Autodesk Fusion 360 part; units mm, degrees
(part 5 of 7)
  line L387 (58.55, -43.6287) -> (58.588, -43.6922)
  line L388 (58.588, -43.6922) -> (58.628, -43.7538)
  line L389 (58.628, -43.7538) -> (58.6706, -43.8129)
  line L390 (58.6706, -43.8129) -> (58.7169, -43.8682)
  line L391 (58.7169, -43.8682) -> (59.0326, -44.185)
  line L392 (59.0326, -44.185) -> (58.8812, -44.34)
  line L393 (58.8812, -44.34) -> (58.734, -44.4991)
  line L394 (58.734, -44.4991) -> (58.5912, -44.6621)
  line L395 (58.5912, -44.6621) -> (58.4529, -44.8289)
  line L396 (58.4529, -44.8289) -> (58.1048, -44.548)
  line L397 (58.1048, -44.548) -> (58.0449, -44.5077)
  line L398 (58.0449, -44.5077) -> (57.9817, -44.4716)
  line L399 (57.9817, -44.4716) -> (57.9163, -44.4382)
  line L400 (57.9163, -44.4382) -> (57.8491, -44.4071)
  line L401 (57.8491, -44.4071) -> (57.7804, -44.3781)
  line L402 (57.7804, -44.3781) -> (57.7102, -44.3509)
  line L403 (57.7102, -44.3509) -> (57.6387, -44.3254)
  line L404 (57.6387, -44.3254) -> (57.566, -44.3017)
  line L405 (57.566, -44.3017) -> (57.4922, -44.2795)
  line L406 (57.4922, -44.2795) -> (57.4173, -44.2588)
  line L407 (57.4173, -44.2588) -> (57.3414, -44.2397)
  line L408 (57.3414, -44.2397) -> (57.2644, -44.222)
  line L409 (57.2644, -44.222) -> (57.1855, -44.3275)
  line L410 (57.1855, -44.3275) -> (57.108, -44.4341)
  line L411 (57.108, -44.4341) -> (57.032, -44.5418)
  line L412 (57.032, -44.5418) -> (57.0726, -44.6095)
  line L413 (57.0726, -44.6095) -> (57.1143, -44.6758)
  line L414 (57.1143, -44.6758) -> (57.1571, -44.7407)
  line L415 (57.1571, -44.7407) -> (57.201, -44.804)
  line L416 (57.201, -44.804) -> (57.2461, -44.8658)
  line L417 (57.2461, -44.8658) -> (57.2924, -44.9259)
  line L418 (57.2924, -44.9259) -> (57.3399, -44.9843)
  line L419 (57.3399, -44.9843) -> (57.3888, -45.0407)
  line L420 (57.3888, -45.0407) -> (57.4392, -45.095)
  line L421 (57.4392, -45.095) -> (57.4911, -45.1469)
  line L422 (57.4911, -45.1469) -> (57.545, -45.1958)
  line L423 (57.545, -45.1958) -> (57.6018, -45.2403)
  line L424 (57.6018, -45.2403) -> (57.9765, -45.4845)
  line L425 (57.9765, -45.4845) -> (57.8606, -45.6677)
  line L426 (57.8606, -45.6677) -> (57.7497, -45.8538)
  line L427 (57.7497, -45.8538) -> (57.6439, -46.0429)
  line L428 (57.6439, -46.0429) -> (57.5433, -46.2348)
  line L429 (57.5433, -46.2348) -> (57.1444, -46.0325)
  line L430 (57.1444, -46.0325) -> (57.0775, -46.0056)
  line L431 (57.0775, -46.0056) -> (57.0082, -45.9834)
  line L432 (57.0082, -45.9834) -> (56.9372, -45.9643)
  line L433 (56.9372, -45.9643) -> (56.8651, -45.9479)
  line L434 (56.8651, -45.9479) -> (56.7918, -45.9337)
  line L435 (56.7918, -45.9337) -> (56.7175, -45.9217)
  line L436 (56.7175, -45.9217) -> (56.6423, -45.9117)
  line L437 (56.6423, -45.9117) -> (56.5662, -45.9035)
  line L438 (56.5662, -45.9035) -> (56.4894, -45.8972)
  line L439 (56.4894, -45.8972) -> (56.4118, -45.8926)
  line L440 (56.4118, -45.8926) -> (56.3336, -45.8896)
  line L441 (56.3336, -45.8896) -> (56.2547, -45.8883)
  line L442 (56.2547, -45.8883) -> (56.1994, -46.0079)
  line L443 (56.1994, -46.0079) -> (56.1458, -46.1283)
  line L444 (56.1458, -46.1283) -> (56.0939, -46.2495)
  line L445 (56.0939, -46.2495) -> (56.1476, -46.3073)
  line L446 (56.1476, -46.3073) -> (56.2022, -46.3634)
  line L447 (56.2022, -46.3634) -> (56.2575, -46.418)
  line L448 (56.2575, -46.418) -> (56.3137, -46.4708)
  line L449 (56.3137, -46.4708) -> (56.3706, -46.5219)
  line L450 (56.3706, -46.5219) -> (56.4284, -46.5711)
  line L451 (56.4284, -46.5711) -> (56.487, -46.6182)
  line L452 (56.487, -46.6182) -> (56.5465, -46.6633)
  line L453 (56.5465, -46.6633) -> (56.6071, -46.7059)
  line L454 (56.6071, -46.7059) -> (56.6687, -46.7458)
  line L455 (56.6687, -46.7458) -> (56.7316, -46.7825)
  line L456 (56.7316, -46.7825) -> (56.7964, -46.8142)
  line L457 (56.7964, -46.8142) -> (57.2136, -46.9753)
  line L458 (57.2136, -46.9753) -> (57.1384, -47.1784)
  line L459 (57.1384, -47.1784) -> (57.0686, -47.3836)
  line L460 (57.0686, -47.3836) -> (57.0045, -47.5906)
  line L461 (57.0045, -47.5906) -> (56.9459, -47.7992)
  line L462 (56.9459, -47.7992) -> (56.5137, -47.6842)
  line L463 (56.5137, -47.6842) -> (56.4426, -47.6718)
  line L464 (56.4426, -47.6718) -> (56.3702, -47.6645)
  line L465 (56.3702, -47.6645) -> (56.2969, -47.6606)
  line L466 (56.2969, -47.6606) -> (56.2228, -47.6595)
  line L467 (56.2228, -47.6595) -> (56.1482, -47.6609)
  line L468 (56.1482, -47.6609) -> (56.0731, -47.6646)
  line L469 (56.0731, -47.6646) -> (55.9974, -47.6705)
  line L470 (55.9974, -47.6705) -> (55.9213, -47.6783)
  line L471 (55.9213, -47.6783) -> (55.8449, -47.6881)
  line L472 (55.8449, -47.6881) -> (55.768, -47.6997)
  line L473 (55.768, -47.6997) -> (55.6909, -47.713)
  line L474 (55.6909, -47.713) -> (55.6134, -47.7282)
  line L475 (55.6134, -47.7282) -> (55.5842, -47.8567)
  line L476 (55.5842, -47.8567) -> (55.5568, -47.9856)
  line L477 (55.5568, -47.9856) -> (55.5312, -48.1149)
  line L478 (55.5312, -48.1149) -> (55.5958, -48.1602)
  line L479 (55.5958, -48.1602) -> (55.6609, -48.2038)
  line L480 (55.6609, -48.2038) -> (55.7263, -48.2457)
  line L481 (55.7263, -48.2457) -> (55.7922, -48.2857)
  line L482 (55.7922, -48.2857) -> (55.8585, -48.3238)
  line L483 (55.8585, -48.3238) -> (55.9253, -48.3599)
  line L484 (55.9253, -48.3599) -> (55.9924, -48.3938)
  line L485 (55.9924, -48.3938) -> (56.06, -48.4255)
  line L486 (56.06, -48.4255) -> (56.1281, -48.4546)
  line L487 (56.1281, -48.4546) -> (56.1967, -48.4809)
  line L488 (56.1967, -48.4809) -> (56.2658, -48.5037)
  line L489 (56.2658, -48.5037) -> (56.3358, -48.5212)
  line L490 (56.3358, -48.5212) -> (56.7774, -48.592)
  line L491 (56.7774, -48.592) -> (56.746, -48.8064)
  line L492 (56.746, -48.8064) -> (56.7205, -49.0216)
  line L493 (56.7205, -49.0216) -> (56.7007, -49.2373)
  line L494 (56.7007, -49.2373) -> (56.6868, -49.4536)
  line L495 (56.6868, -49.4536) -> (56.2402, -49.431)
  line L496 (56.2402, -49.431) -> (56.1681, -49.4336)
  line L497 (56.1681, -49.4336) -> (56.0957, -49.4415)
  line L498 (56.0957, -49.4415) -> (56.0232, -49.4529)
  line L499 (56.0232, -49.4529) -> (55.9505, -49.4673)
  line L500 (55.9505, -49.4673) -> (55.8778, -49.4842)
  line L501 (55.8778, -49.4842) -> (55.8051, -49.5034)
  line L502 (55.8051, -49.5034) -> (55.7323, -49.5249)
  line L503 (55.7323, -49.5249) -> (55.6595, -49.5483)
  line L504 (55.6595, -49.5483) -> (55.5867, -49.5738)
  line L505 (55.5867, -49.5738) -> (55.514, -49.6011)
  line L506 (55.514, -49.6011) -> (55.4413, -49.6302)
  line L507 (55.4413, -49.6302) -> (55.3687, -49.6611)
  line L508 (55.3687, -49.6611) -> (55.3668, -49.7929)
  line L509 (55.3668, -49.7929) -> (55.3668, -49.9247)
  line L510 (55.3668, -49.9247) -> (55.3687, -50.0565)
  line L511 (55.3687, -50.0565) -> (55.4413, -50.0874)
  line L512 (55.4413, -50.0874) -> (55.514, -50.1166)
  line L513 (55.514, -50.1166) -> (55.5867, -50.1439)
  line L514 (55.5867, -50.1439) -> (55.6595, -50.1693)
  line L515 (55.6595, -50.1693) -> (55.7323, -50.1928)
  line L516 (55.7323, -50.1928) -> (55.8051, -50.2142)
  line L517 (55.8051, -50.2142) -> (55.8778, -50.2335)
  line L518 (55.8778, -50.2335) -> (55.9505, -50.2504)
  line L519 (55.9505, -50.2504) -> (56.0232, -50.2647)
  line L520 (56.0232, -50.2647) -> (56.0957, -50.2762)
  line L521 (56.0957, -50.2762) -> (56.1681, -50.2841)
  line L522 (56.1681, -50.2841) -> (56.2402, -50.2867)
  line L523 (56.2402, -50.2867) -> (56.6868, -50.2641)
  line L524 (56.6868, -50.2641) -> (56.7007, -50.4803)
  line L525 (56.7007, -50.4803) -> (56.7205, -50.6961)
  line L526 (56.7205, -50.6961) -> (56.746, -50.9113)
  line L527 (56.746, -50.9113) -> (56.7774, -51.1257)
  line L528 (56.7774, -51.1257) -> (56.3358, -51.1964)
  line L529 (56.3358, -51.1964) -> (56.2658, -51.214)
  line L530 (56.2658, -51.214) -> (56.1967, -51.2368)
  line L531 (56.1967, -51.2368) -> (56.1281, -51.263)
  line L532 (56.1281, -51.263) -> (56.06, -51.2922)
  line L533 (56.06, -51.2922) -> (55.9924, -51.3238)
  line L534 (55.9924, -51.3238) -> (55.9253, -51.3578)
  line L535 (55.9253, -51.3578) -> (55.8585, -51.3939)
  line L536 (55.8585, -51.3939) -> (55.7922, -51.432)
  line L537 (55.7922, -51.432) -> (55.7263, -51.472)
  line L538 (55.7263, -51.472) -> (55.6609, -51.5138)
  line L539 (55.6609, -51.5138) -> (55.5958, -51.5574)
  line L540 (55.5958, -51.5574) -> (55.5312, -51.6028)
  line L541 (55.5312, -51.6028) -> (55.5568, -51.7321)
  line L542 (55.5568, -51.7321) -> (55.5842, -51.861)
  line L543 (55.5842, -51.861) -> (55.6134, -51.9895)
  line L544 (55.6134, -51.9895) -> (55.6909, -52.0046)
  line L545 (55.6909, -52.0046) -> (55.768, -52.018)
  line L546 (55.768, -52.018) -> (55.8449, -52.0296)
  line L547 (55.8449, -52.0296) -> (55.9213, -52.0394)
  line L548 (55.9213, -52.0394) -> (55.9974, -52.0472)
  line L549 (55.9974, -52.0472) -> (56.0731, -52.053)
  line L550 (56.0731, -52.053) -> (56.1482, -52.0567)
  line L551 (56.1482, -52.0567) -> (56.2228, -52.0582)
  line L552 (56.2228, -52.0582) -> (56.2969, -52.0571)
  line L553 (56.2969, -52.0571) -> (56.3702, -52.0532)
  line L554 (56.3702, -52.0532) -> (56.4426, -52.0459)
  line L555 (56.4426, -52.0459) -> (56.5137, -52.0335)
  line L556 (56.5137, -52.0335) -> (56.9459, -51.9185)
  line L557 (56.9459, -51.9185) -> (57.0045, -52.1271)
  line L558 (57.0045, -52.1271) -> (57.0686, -52.3341)
  line L559 (57.0686, -52.3341) -> (57.1384, -52.5392)
  line L560 (57.1384, -52.5392) -> (57.2136, -52.7424)
  line L561 (57.2136, -52.7424) -> (56.7964, -52.9034)
  line L562 (56.7964, -52.9034) -> (56.7316, -52.9352)
  line L563 (56.7316, -52.9352) -> (56.6687, -52.9718)
  line L564 (56.6687, -52.9718) -> (56.6071, -53.0118)
  line L565 (56.6071, -53.0118) -> (56.5465, -53.0544)
  line L566 (56.5465, -53.0544) -> (56.487, -53.0994)
  line L567 (56.487, -53.0994) -> (56.4284, -53.1466)
  line L568 (56.4284, -53.1466) -> (56.3706, -53.1958)
  line L569 (56.3706, -53.1958) -> (56.3137, -53.2468)
  line L570 (56.3137, -53.2468) -> (56.2575, -53.2997)
  line L571 (56.2575, -53.2997) -> (56.2022, -53.3542)
  line L572 (56.2022, -53.3542) -> (56.1476, -53.4104)
  line L573 (56.1476, -53.4104) -> (56.0939, -53.4682)
  line L574 (56.0939, -53.4682) -> (56.1458, -53.5893)
  line L575 (56.1458, -53.5893) -> (56.1994, -53.7097)
  line L576 (56.1994, -53.7097) -> (56.2547, -53.8294)
  line L577 (56.2547, -53.8294) -> (56.3336, -53.828)
  line L578 (56.3336, -53.828) -> (56.4118, -53.8251)
  line L579 (56.4118, -53.8251) -> (56.4894, -53.8205)
  line L580 (56.4894, -53.8205) -> (56.5662, -53.8141)
  line L581 (56.5662, -53.8141) -> (56.6423, -53.806)
  line L582 (56.6423, -53.806) -> (56.7175, -53.7959)
  line L583 (56.7175, -53.7959) -> (56.7918, -53.7839)
  line L584 (56.7918, -53.7839) -> (56.8651, -53.7698)
  line L585 (56.8651, -53.7698) -> (56.9372, -53.7534)
  line L586 (56.9372, -53.7534) -> (57.0082, -53.7343)
  line L587 (57.0082, -53.7343) -> (57.0775, -53.7121)
  line L588 (57.0775, -53.7121) -> (57.1444, -53.6852)
  line L589 (57.1444, -53.6852) -> (57.5433, -53.4828)
  line L590 (57.5433, -53.4828) -> (57.6439, -53.6747)
  line L591 (57.6439, -53.6747) -> (57.7497, -53.8638)
  line L592 (57.7497, -53.8638) -> (57.8606, -54.05)
  line L593 (57.8606, -54.05) -> (57.9765, -54.2331)
  line L594 (57.9765, -54.2331) -> (57.6018, -54.4773)
  line L595 (57.6018, -54.4773) -> (57.545, -54.5219)
  line L596 (57.545, -54.5219) -> (57.4911, -54.5708)
  line L597 (57.4911, -54.5708) -> (57.4392, -54.6227)
  line L598 (57.4392, -54.6227) -> (57.3888, -54.677)
  line L599 (57.3888, -54.677) -> (57.3399, -54.7334)
  line L600 (57.3399, -54.7334) -> (57.2924, -54.7917)
  line L601 (57.2924, -54.7917) -> (57.2461, -54.8518)
  line L602 (57.2461, -54.8518) -> (57.201, -54.9136)
  line L603 (57.201, -54.9136) -> (57.1571, -54.977)
  line L604 (57.1571, -54.977) -> (57.1143, -55.0418)
  line L605 (57.1143, -55.0418) -> (57.0726, -55.1081)
  line L606 (57.0726, -55.1081) -> (57.032, -55.1758)
  line L607 (57.032, -55.1758) -> (57.108, -55.2835)
  line L608 (57.108, -55.2835) -> (57.1855, -55.3902)
  line L609 (57.1855, -55.3902) -> (57.2644, -55.4957)
  line L610 (57.2644, -55.4957) -> (57.3414, -55.478)
  line L611 (57.3414, -55.478) -> (57.4173, -55.4588)
  line L612 (57.4173, -55.4588) -> (57.4922, -55.4382)
  line L613 (57.4922, -55.4382) -> (57.566, -55.416)
  line L614 (57.566, -55.416) -> (57.6387, -55.3922)
  line L615 (57.6387, -55.3922) -> (57.7102, -55.3668)
  line L616 (57.7102, -55.3668) -> (57.7804, -55.3396)
  line L617 (57.7804, -55.3396) -> (57.8491, -55.3105)
  line L618 (57.8491, -55.3105) -> (57.9163, -55.2794)
  line L619 (57.9163, -55.2794) -> (57.9817, -55.2461)
  line L620 (57.9817, -55.2461) -> (58.0449, -55.2099)
  line L621 (58.0449, -55.2099) -> (58.1048, -55.1697)
  line L622 (58.1048, -55.1697) -> (58.4529, -54.8888)
  line L623 (58.4529, -54.8888) -> (58.5912, -55.0556)
  line L624 (58.5912, -55.0556) -> (58.734, -55.2186)
  line L625 (58.734, -55.2186) -> (58.8812, -55.3776)
  line L626 (58.8812, -55.3776) -> (59.0326, -55.5326)
  line L627 (59.0326, -55.5326) -> (58.7169, -55.8494)
  line L628 (58.7169, -55.8494) -> (58.6706, -55.9048)
  line L629 (58.6706, -55.9048) -> (58.628, -55.9639)
  line L630 (58.628, -55.9639) -> (58.588, -56.0254)
  line L631 (58.588, -56.0254) -> (58.55, -56.089)
  line L632 (58.55, -56.089) -> (58.514, -56.1543)
  line L633 (58.514, -56.1543) -> (58.4796, -56.2213)
  line L634 (58.4796, -56.2213) -> (58.4468, -56.2897)
  line L635 (58.4468, -56.2897) -> (58.4156, -56.3595)
  line L636 (58.4156, -56.3595) -> (58.3858, -56.4306)
  line L637 (58.3858, -56.4306) -> (58.3574, -56.5029)
  line L638 (58.3574, -56.5029) -> (58.3304, -56.5765)
  line L639 (58.3304, -56.5765) -> (58.3048, -56.6511)
  line L640 (58.3048, -56.6511) -> (58.4015, -56.7407)
  line L641 (58.4015, -56.7407) -> (58.4994, -56.8289)
  line L642 (58.4994, -56.8289) -> (58.5986, -56.9157)
  line L643 (58.5986, -56.9157) -> (58.6702, -56.8824)
  line L644 (58.6702, -56.8824) -> (58.7405, -56.8478)
  line L645 (58.7405, -56.8478) -> (58.8094, -56.8121)
  line L646 (58.8094, -56.8121) -> (58.877, -56.775)
  line L647 (58.877, -56.775) -> (58.9432, -56.7366)
  line L648 (58.9432, -56.7366) -> (59.0078, -56.6969)
  line L649 (59.0078, -56.6969) -> (59.0708, -56.6557)
  line L650 (59.0708, -56.6557) -> (59.132, -56.613)
  line L651 (59.132, -56.613) -> (59.1913, -56.5686)
  line L652 (59.1913, -56.5686) -> (59.2483, -56.5224)
  line L653 (59.2483, -56.5224) -> (59.3026, -56.4739)
  line L654 (59.3026, -56.4739) -> (59.3528, -56.422)
  line L655 (59.3528, -56.422) -> (59.6349, -56.075)
  line L656 (59.6349, -56.075) -> (59.8049, -56.2093)
  line L657 (59.8049, -56.2093) -> (59.9784, -56.3391)
  line L658 (59.9784, -56.3391) -> (60.1554, -56.464)
  line L659 (60.1554, -56.464) -> (60.3358, -56.5842)
  line L660 (60.3358, -56.5842) -> (60.0928, -56.9597)
  line L661 (60.0928, -56.9597) -> (60.0591, -57.0235)
  line L662 (60.0591, -57.0235) -> (60.0297, -57.0901)
  line L663 (60.0297, -57.0901) -> (60.0034, -57.1586)
  line L664 (60.0034, -57.1586) -> (59.9795, -57.2287)
  line L665 (59.9795, -57.2287) -> (59.9578, -57.3001)
  line L666 (59.9578, -57.3001) -> (59.9381, -57.3727)
  line L667 (59.9381, -57.3727) -> (59.9202, -57.4465)
  line L668 (59.9202, -57.4465) -> (59.9042, -57.5213)
  line L669 (59.9042, -57.5213) -> (59.8898, -57.597)
  line L670 (59.8898, -57.597) -> (59.8771, -57.6737)
  line L671 (59.8771, -57.6737) -> (59.866, -57.7512)
  line L672 (59.866, -57.7512) -> (59.8564, -57.8295)
  line L673 (59.8564, -57.8295) -> (59.9696, -57.897)
  line L674 (59.9696, -57.897) -> (60.0838, -57.9629)
  line L675 (60.0838, -57.9629) -> (60.1988, -58.0272)
  line L676 (60.1988, -58.0272) -> (60.2619, -57.9798)
  line L677 (60.2619, -57.9798) -> (60.3235, -57.9314)
  line L678 (60.3235, -57.9314) -> (60.3835, -57.882)
  line L679 (60.3835, -57.882) -> (60.4419, -57.8317)
  line L680 (60.4419, -57.8317) -> (60.4987, -57.7805)
  line L681 (60.4987, -57.7805) -> (60.5536, -57.7281)
  line L682 (60.5536, -57.7281) -> (60.6067, -57.6748)
  line L683 (60.6067, -57.6748) -> (60.6577, -57.6202)
  line L684 (60.6577, -57.6202) -> (60.7064, -57.5645)
  line L685 (60.7064, -57.5645) -> (60.7526, -57.5074)
  line L686 (60.7526, -57.5074) -> (60.7956, -57.4487)
  line L687 (60.7956, -57.4487) -> (60.8339, -57.3876)
  line L688 (60.8339, -57.3876) -> (61.0377, -56.9894)
  line L689 (61.0377, -56.9894) -> (61.2319, -57.0855)
  line L690 (61.2319, -57.0855) -> (61.4286, -57.1763)
  line L691 (61.4286, -57.1763) -> (61.6278, -57.2618)
  line L692 (61.6278, -57.2618) -> (61.8291, -57.3418)
  line L693 (61.8291, -57.3418) -> (61.6696, -57.7596)
  line L694 (61.6696, -57.7596) -> (61.6498, -57.829)
  line L695 (61.6498, -57.829) -> (61.635, -57.9003)
  line L696 (61.635, -57.9003) -> (61.6234, -57.9728)
  line L697 (61.6234, -57.9728) -> (61.6146, -58.0463)
  line L698 (61.6146, -58.0463) -> (61.6082, -58.1207)
  line L699 (61.6082, -58.1207) -> (61.604, -58.1958)
  line L700 (61.604, -58.1958) -> (61.6019, -58.2717)
  line L701 (61.6019, -58.2717) -> (61.6018, -58.3481)
  line L702 (61.6018, -58.3481) -> (61.6035, -58.4252)
  line L703 (61.6035, -58.4252) -> (61.607, -58.5028)
  line L704 (61.607, -58.5028) -> (61.6122, -58.581)
  line L705 (61.6122, -58.581) -> (61.6192, -58.6596)
  line L706 (61.6192, -58.6596) -> (61.7439, -58.7021)
  line L707 (61.7439, -58.7021) -> (61.8693, -58.7428)
  line L708 (61.8693, -58.7428) -> (61.9952, -58.7818)
  line L709 (61.9952, -58.7818) -> (62.047, -58.7222)
  line L710 (62.047, -58.7222) -> (62.0972, -58.6621)
  line L711 (62.0972, -58.6621) -> (62.1457, -58.6014)
  line L712 (62.1457, -58.6014) -> (62.1924, -58.54)
  line L713 (62.1924, -58.54) -> (62.2372, -58.4781)
  line L714 (62.2372, -58.4781) -> (62.28, -58.4155)
  line L715 (62.28, -58.4155) -> (62.3208, -58.3522)
  line L716 (62.3208, -58.3522) -> (62.3594, -58.2883)
  line L717 (62.3594, -58.2883) -> (62.3955, -58.2237)
  line L718 (62.3955, -58.2237) -> (62.4288, -58.1582)
  line L719 (62.4288, -58.1582) -> (62.4586, -58.0918)
  line L720 (62.4586, -58.0918) -> (62.4834, -58.0241)
  line L721 (62.4834, -58.0241) -> (62.5999, -57.5923)
  line L722 (62.5999, -57.5923) -> (62.8099, -57.6459)
  line L723 (62.8099, -57.6459) -> (63.0212, -57.6938)
  line L724 (63.0212, -57.6938) -> (63.2338, -57.736)
  line L725 (63.2338, -57.736) -> (63.4474, -57.7724)
  line L726 (63.4474, -57.7724) -> (63.3782, -58.2142)
  line L727 (63.3782, -58.2142) -> (63.3733, -58.2862)
  line L728 (63.3733, -58.2862) -> (63.3736, -58.359)
  line L729 (63.3736, -58.359) -> (63.3773, -58.4324)
  line L730 (63.3773, -58.4324) -> (63.384, -58.5061)
  line L731 (63.384, -58.5061) -> (63.3932, -58.5802)
  line L732 (63.3932, -58.5802) -> (63.4048, -58.6545)
  line L733 (63.4048, -58.6545) -> (63.4185, -58.7292)
  line L734 (63.4185, -58.7292) -> (63.4342, -58.804)
  line L735 (63.4342, -58.804) -> (63.4519, -58.879)
  line L736 (63.4519, -58.879) -> (63.4715, -58.9542)
  line L737 (63.4715, -58.9542) -> (63.4929, -59.0296)
  line L738 (63.4929, -59.0296) -> (63.516, -59.105)
  line L739 (63.516, -59.105) -> (63.6469, -59.1207)
  line L740 (63.6469, -59.1207) -> (63.7779, -59.1344)
  line L741 (63.7779, -59.1344) -> (63.9092, -59.1464)
  line L742 (63.9092, -59.1464) -> (63.9475, -59.0774)
  line L743 (63.9475, -59.0774) -> (63.9841, -59.0081)
  line L744 (63.9841, -59.0081) -> (64.0189, -58.9386)
  line L745 (64.0189, -58.9386) -> (64.0518, -58.8689)
  line L746 (64.0518, -58.8689) -> (64.0827, -58.799)
  line L747 (64.0827, -58.799) -> (64.1117, -58.7288)
  line L748 (64.1117, -58.7288) -> (64.1384, -58.6585)
  line L749 (64.1384, -58.6585) -> (64.1628, -58.588)
  line L750 (64.1628, -58.588) -> (64.1847, -58.5172)
  line L751 (64.1847, -58.5172) -> (64.2036, -58.4463)
  line L752 (64.2036, -58.4463) -> (64.2191, -58.3751)
  line L753 (64.2191, -58.3751) -> (64.2292, -58.3037)
  line L754 (64.2292, -58.3037) -> (64.2534, -57.8571)
  line L755 (64.2534, -57.8571) -> (64.4699, -57.8659)
  line L756 (64.4699, -57.8659) -> (64.6866, -57.8688)
  line L757 (64.6866, -57.8688) -> (64.9033, -57.8659)
  line L758 (64.9033, -57.8659) -> (65.1198, -57.8571)
  line L759 (65.1198, -57.8571) -> (65.1439, -58.3037)
  line L760 (65.1439, -58.3037) -> (65.1541, -58.3751)
  line L761 (65.1541, -58.3751) -> (65.1695, -58.4463)
  line L762 (65.1695, -58.4463) -> (65.1885, -58.5172)
  line L763 (65.1885, -58.5172) -> (65.2103, -58.588)
  line L764 (65.2103, -58.588) -> (65.2348, -58.6585)
  line L765 (65.2348, -58.6585) -> (65.2615, -58.7288)
  line L766 (65.2615, -58.7288) -> (65.2904, -58.799)
  line L767 (65.2904, -58.799) -> (65.3214, -58.8689)
  line L768 (65.3214, -58.8689) -> (65.3543, -58.9386)
  line L769 (65.3543, -58.9386) -> (65.3891, -59.0081)
  line L770 (65.3891, -59.0081) -> (65.4256, -59.0774)
  line L771 (65.4256, -59.0774) -> (65.464, -59.1464)
  line L772 (65.464, -59.1464) -> (65.5952, -59.1344)
  line L773 (65.5952, -59.1344) -> (65.7263, -59.1207)
  line L774 (65.7263, -59.1207) -> (65.8572, -59.105)
  line L775 (65.8572, -59.105) -> (65.8803, -59.0296)
  line L776 (65.8803, -59.0296) -> (65.9017, -58.9542)
  line L777 (65.9017, -58.9542) -> (65.9213, -58.879)
  line L778 (65.9213, -58.879) -> (65.939, -58.804)
  line L779 (65.939, -58.804) -> (65.9547, -58.7292)
  line L780 (65.9547, -58.7292) -> (65.9684, -58.6545)
  line L781 (65.9684, -58.6545) -> (65.9799, -58.5802)
  line L782 (65.9799, -58.5802) -> (65.9892, -58.5061)
  line L783 (65.9892, -58.5061) -> (65.9958, -58.4324)
  line L784 (65.9958, -58.4324) -> (65.9996, -58.359)
  line L785 (65.9996, -58.359) -> (65.9999, -58.2862)
  line L786 (65.9999, -58.2862) -> (65.995, -58.2142)
  line L787 (65.995, -58.2142) -> (65.9258, -57.7724)
  line L788 (65.9258, -57.7724) -> (66.1394, -57.736)
  line L789 (66.1394, -57.736) -> (66.352, -57.6938)
  line L790 (66.352, -57.6938) -> (66.5633, -57.6459)
  line L791 (66.5633, -57.6459) -> (66.7732, -57.5923)
  line L792 (66.7732, -57.5923) -> (66.8897, -58.0241)
  line L793 (66.8897, -58.0241) -> (66.9145, -58.0918)
  line L794 (66.9145, -58.0918) -> (66.9444, -58.1582)
  line L795 (66.9444, -58.1582) -> (66.9777, -58.2237)
  line L796 (66.9777, -58.2237) -> (67.0138, -58.2883)
  line L797 (67.0138, -58.2883) -> (67.0523, -58.3522)
  line L798 (67.0523, -58.3522) -> (67.0931, -58.4155)
  line L799 (67.0931, -58.4155) -> (67.136, -58.4781)
  line L800 (67.136, -58.4781) -> (67.1808, -58.54)
  line L801 (67.1808, -58.54) -> (67.2275, -58.6014)
  line L802 (67.2275, -58.6014) -> (67.276, -58.6621)
  line L803 (67.276, -58.6621) -> (67.3261, -58.7222)
  line L804 (67.3261, -58.7222) -> (67.378, -58.7818)
  line L805 (67.378, -58.7818) -> (67.5039, -58.7428)
  line L806 (67.5039, -58.7428) -> (67.6292, -58.7021)
  line L807 (67.6292, -58.7021) -> (67.754, -58.6596)
  line L808 (67.754, -58.6596) -> (67.7609, -58.581)
  line L809 (67.7609, -58.581) -> (67.7662, -58.5028)
  line L810 (67.7662, -58.5028) -> (67.7697, -58.4252)
  line L811 (67.7697, -58.4252) -> (67.7714, -58.3481)
  line L812 (67.7714, -58.3481) -> (67.7712, -58.2717)
  line L813 (67.7712, -58.2717) -> (67.7691, -58.1958)
  line L814 (67.7691, -58.1958) -> (67.7649, -58.1207)
  line L815 (67.7649, -58.1207) -> (67.7586, -58.0463)
  line L816 (67.7586, -58.0463) -> (67.7498, -57.9728)
  line L817 (67.7498, -57.9728) -> (67.7382, -57.9003)
  line L818 (67.7382, -57.9003) -> (67.7234, -57.829)
  line L819 (67.7234, -57.829) -> (67.7036, -57.7596)
  line L820 (67.7036, -57.7596) -> (67.5441, -57.3418)
  line L821 (67.5441, -57.3418) -> (67.7454, -57.2618)
  line L822 (67.7454, -57.2618) -> (67.9445, -57.1763)
  line L823 (67.9445, -57.1763) -> (68.1413, -57.0855)
  line L824 (68.1413, -57.0855) -> (68.3355, -56.9894)
  line L825 (68.3355, -56.9894) -> (68.5392, -57.3876)
  line L826 (68.5392, -57.3876) -> (68.5776, -57.4487)
  line L827 (68.5776, -57.4487) -> (68.6206, -57.5074)
  line L828 (68.6206, -57.5074) -> (68.6668, -57.5645)
  line L829 (68.6668, -57.5645) -> (68.7155, -57.6202)
  line L830 (68.7155, -57.6202) -> (68.7665, -57.6748)
  line L831 (68.7665, -57.6748) -> (68.8196, -57.7281)
  line L832 (68.8196, -57.7281) -> (68.8745, -57.7805)
  line L833 (68.8745, -57.7805) -> (68.9312, -57.8317)
  line L834 (68.9312, -57.8317) -> (68.9897, -57.882)
  line L835 (68.9897, -57.882) -> (69.0497, -57.9314)
  line L836 (69.0497, -57.9314) -> (69.1113, -57.9798)
  line L837 (69.1113, -57.9798) -> (69.1743, -58.0272)
  line L838 (69.1743, -58.0272) -> (69.2894, -57.9629)
  line L839 (69.2894, -57.9629) -> (69.4035, -57.897)
  line L840 (69.4035, -57.897) -> (69.5167, -57.8295)
  line L841 (69.5167, -57.8295) -> (69.5072, -57.7512)
  line L842 (69.5072, -57.7512) -> (69.4961, -57.6737)
  line L843 (69.4961, -57.6737) -> (69.4834, -57.597)
  line L844 (69.4834, -57.597) -> (69.469, -57.5213)
  line L845 (69.469, -57.5213) -> (69.453, -57.4465)
  line L846 (69.453, -57.4465) -> (69.4351, -57.3727)
  line L847 (69.4351, -57.3727) -> (69.4154, -57.3001)
  line L848 (69.4154, -57.3001) -> (69.3937, -57.2287)
  line L849 (69.3937, -57.2287) -> (69.3698, -57.1586)
  line L850 (69.3698, -57.1586) -> (69.3435, -57.0901)
  line L851 (69.3435, -57.0901) -> (69.3141, -57.0235)
  line L852 (69.3141, -57.0235) -> (69.2803, -56.9597)
  line L853 (69.2803, -56.9597) -> (69.0374, -56.5842)
  line L854 (69.0374, -56.5842) -> (69.2177, -56.464)
  line L855 (69.2177, -56.464) -> (69.3947, -56.3391)
  line L856 (69.3947, -56.3391) -> (69.5683, -56.2093)
  line L857 (69.5683, -56.2093) -> (69.7383, -56.075)
  line L858 (69.7383, -56.075) -> (70.0204, -56.422)
  line L859 (70.0204, -56.422) -> (70.0706, -56.4739)
  line L860 (70.0706, -56.4739) -> (70.1249, -56.5224)
  line L861 (70.1249, -56.5224) -> (70.1819, -56.5686)
  line L862 (70.1819, -56.5686) -> (70.2412, -56.613)
  line L863 (70.2412, -56.613) -> (70.3024, -56.6557)
  line L864 (70.3024, -56.6557) -> (70.3654, -56.6969)
  line L865 (70.3654, -56.6969) -> (70.43, -56.7366)
  line L866 (70.43, -56.7366) -> (70.4961, -56.775)
  line L867 (70.4961, -56.775) -> (70.5637, -56.8121)
  line L868 (70.5637, -56.8121) -> (70.6327, -56.8478)
  line L869 (70.6327, -56.8478) -> (70.703, -56.8824)
  line L870 (70.703, -56.8824) -> (70.7746, -56.9157)
  line L871 (70.7746, -56.9157) -> (70.8738, -56.8289)
  line L872 (70.8738, -56.8289) -> (70.9717, -56.7407)
  line L873 (70.9717, -56.7407) -> (71.0684, -56.6511)
  line L874 (71.0684, -56.6511) -> (71.0428, -56.5765)
  line L875 (71.0428, -56.5765) -> (71.0158, -56.5029)
  line L876 (71.0158, -56.5029) -> (70.9874, -56.4306)
  line L877 (70.9874, -56.4306) -> (70.9576, -56.3595)
  line L878 (70.9576, -56.3595) -> (70.9264, -56.2897)
  line L879 (70.9264, -56.2897) -> (70.8936, -56.2213)
  line L880 (70.8936, -56.2213) -> (70.8592, -56.1543)
  line L881 (70.8592, -56.1543) -> (70.8231, -56.089)
  line L882 (70.8231, -56.089) -> (70.7852, -56.0254)
  line L883 (70.7852, -56.0254) -> (70.7452, -55.9639)
  line L884 (70.7452, -55.9639) -> (70.7026, -55.9048)
  line L885 (70.7026, -55.9048) -> (70.6563, -55.8494)
  line L886 (70.6563, -55.8494) -> (70.3406, -55.5326)
  line L887 (70.3406, -55.5326) -> (70.492, -55.3776)
  line L888 (70.492, -55.3776) -> (70.6392, -55.2186)
  line L889 (70.6392, -55.2186) -> (70.782, -55.0556)
  line L890 (70.782, -55.0556) -> (70.9203, -54.8888)
  line L891 (70.9203, -54.8888) -> (71.2684, -55.1697)
  line L892 (71.2684, -55.1697) -> (71.3283, -55.2099)
  line L893 (71.3283, -55.2099) -> (71.3915, -55.2461)
  line L894 (71.3915, -55.2461) -> (71.4569, -55.2794)
  line L895 (71.4569, -55.2794) -> (71.5241, -55.3105)
  line L896 (71.5241, -55.3105) -> (71.5928, -55.3396)
  line L897 (71.5928, -55.3396) -> (71.663, -55.3668)
  line L898 (71.663, -55.3668) -> (71.7345, -55.3922)
  line L899 (71.7345, -55.3922) -> (71.8071, -55.416)
  line L900 (71.8071, -55.416) -> (71.881, -55.4382)
  line L901 (71.881, -55.4382) -> (71.9559, -55.4588)
  line L902 (71.9559, -55.4588) -> (72.0318, -55.478)
  line L903 (72.0318, -55.478) -> (72.1087, -55.4957)
  line L904 (72.1087, -55.4957) -> (72.1877, -55.3902)
  line L905 (72.1877, -55.3902) -> (72.2652, -55.2835)
  line L906 (72.2652, -55.2835) -> (72.3411, -55.1758)
  line L907 (72.3411, -55.1758) -> (72.3005, -55.1081)
  line L908 (72.3005, -55.1081) -> (72.2588, -55.0418)
  line L909 (72.2588, -55.0418) -> (72.2161, -54.977)
  line L910 (72.2161, -54.977) -> (72.1721, -54.9136)
  line L911 (72.1721, -54.9136) -> (72.1271, -54.8518)
  line L912 (72.1271, -54.8518) -> (72.0808, -54.7917)
  line L913 (72.0808, -54.7917) -> (72.0332, -54.7334)
  line L914 (72.0332, -54.7334) -> (71.9843, -54.677)
  line L915 (71.9843, -54.677) -> (71.934, -54.6227)
  line L916 (71.934, -54.6227) -> (71.8821, -54.5708)
  line L917 (71.8821, -54.5708) -> (71.8282, -54.5219)
  line L918 (71.8282, -54.5219) -> (71.7714, -54.4773)
  line L919 (71.7714, -54.4773) -> (71.3967, -54.2331)
  line L920 (71.3967, -54.2331) -> (71.5126, -54.05)
  line L921 (71.5126, -54.05) -> (71.6234, -53.8638)
  line L922 (71.6234, -53.8638) -> (71.7292, -53.6747)
  line L923 (71.7292, -53.6747) -> (71.8299, -53.4828)
  line L924 (71.8299, -53.4828) -> (72.2287, -53.6852)
  line L925 (72.2287, -53.6852) -> (72.2957, -53.7121)
  line L926 (72.2957, -53.7121) -> (72.365, -53.7343)
  line L927 (72.365, -53.7343) -> (72.4359, -53.7534)
  line L928 (72.4359, -53.7534) -> (72.5081, -53.7698)
  line L929 (72.5081, -53.7698) -> (72.5814, -53.7839)
  line L930 (72.5814, -53.7839) -> (72.6557, -53.7959)
  line L931 (72.6557, -53.7959) -> (72.7309, -53.806)
  line L932 (72.7309, -53.806) -> (72.8069, -53.8141)
  line L933 (72.8069, -53.8141) -> (72.8838, -53.8205)
  line L934 (72.8838, -53.8205) -> (72.9613, -53.8251)
  line L935 (72.9613, -53.8251) -> (73.0396, -53.828)
  line L936 (73.0396, -53.828) -> (73.1185, -53.8294)
  line L937 (73.1185, -53.8294) -> (73.1738, -53.7097)
  line L938 (73.1738, -53.7097) -> (73.2274, -53.5893)
  line L939 (73.2274, -53.5893) -> (73.2793, -53.4682)
  line L940 (73.2793, -53.4682) -> (73.2255, -53.4104)
  line L941 (73.2255, -53.4104) -> (73.171, -53.3542)
  line L942 (73.171, -53.3542) -> (73.1156, -53.2997)
  line L943 (73.1156, -53.2997) -> (73.0595, -53.2468)
  line L944 (73.0595, -53.2468) -> (73.0026, -53.1958)
  line L945 (73.0026, -53.1958) -> (72.9448, -53.1466)
  line L946 (72.9448, -53.1466) -> (72.8862, -53.0994)
  line L947 (72.8862, -53.0994) -> (72.8266, -53.0544)
  line L948 (72.8266, -53.0544) -> (72.7661, -53.0118)
  line L949 (72.7661, -53.0118) -> (72.7045, -52.9718)
  line L950 (72.7045, -52.9718) -> (72.6416, -52.9352)
  line L951 (72.6416, -52.9352) -> (72.5768, -52.9034)
  line L952 (72.5768, -52.9034) -> (72.1595, -52.7424)
  line L953 (72.1595, -52.7424) -> (72.2348, -52.5392)
  line L954 (72.2348, -52.5392) -> (72.3045, -52.3341)
  line L955 (72.3045, -52.3341) -> (72.3687, -52.1271)
  line L956 (72.3687, -52.1271) -> (72.4273, -51.9185)
  line L957 (72.4273, -51.9185) -> (72.8595, -52.0335)
  line L958 (72.8595, -52.0335) -> (72.9305, -52.0459)
  line L959 (72.9305, -52.0459) -> (73.003, -52.0532)
  line L960 (73.003, -52.0532) -> (73.0763, -52.0571)
  line L961 (73.0763, -52.0571) -> (73.1503, -52.0582)
  line L962 (73.1503, -52.0582) -> (73.225, -52.0567)
  line L963 (73.225, -52.0567) -> (73.3001, -52.053)
  line L964 (73.3001, -52.053) -> (73.3758, -52.0472)
  line L965 (73.3758, -52.0472) -> (73.4518, -52.0394)
  line L966 (73.4518, -52.0394) -> (73.5283, -52.0296)
  line L967 (73.5283, -52.0296) -> (73.6051, -52.018)
  line L968 (73.6051, -52.018) -> (73.6823, -52.0046)
  line L969 (73.6823, -52.0046) -> (73.7598, -51.9895)
  line L970 (73.7598, -51.9895) -> (73.789, -51.861)
  line L971 (73.789, -51.861) -> (73.8164, -51.7321)
  line L972 (73.8164, -51.7321) -> (73.842, -51.6028)
  line L973 (73.842, -51.6028) -> (73.7774, -51.5574)
  line L974 (73.7774, -51.5574) -> (73.7123, -51.5138)
  line L975 (73.7123, -51.5138) -> (73.6468, -51.472)
  line L976 (73.6468, -51.472) -> (73.5809, -51.432)
  line L977 (73.5809, -51.432) -> (73.5146, -51.3939)
  line L978 (73.5146, -51.3939) -> (73.4479, -51.3578)
  line L979 (73.4479, -51.3578) -> (73.3807, -51.3238)
  line L980 (73.3807, -51.3238) -> (73.3131, -51.2922)
  line L981 (73.3131, -51.2922) -> (73.2451, -51.263)
  line L982 (73.2451, -51.263) -> (73.1765, -51.2368)
  line L983 (73.1765, -51.2368) -> (73.1074, -51.214)
  line L984 (73.1074, -51.214) -> (73.0374, -51.1964)
  line L985 (73.0374, -51.1964) -> (72.5958, -51.1257)
  line L986 (72.5958, -51.1257) -> (72.6271, -50.9113)
  line L987 (72.6271, -50.9113) -> (72.6527, -50.6961)
  line L988 (72.6527, -50.6961) -> (72.6724, -50.4803)
  line L989 (72.6724, -50.4803) -> (72.6863, -50.2641)
  circle A0 centre (64.6866, -49.8588) radius 1.5
extrude "Extrude1'''" add sketch "Sketch1 (4)" along normal blind 2 separate body makes body 8 in component "CT idler 3"
ref_plane "WorkPlane2" through (0, 0, 43.4) normal (0, 0, 1) x (1, 0, 0) in component "CT idler 3"
sketch "Sketch2 (3)" plane through (0, 0, 43.4) normal (0, 0, 1) x (1, 0, 0) in component "CT idler 3"
  line L0 (67.7406, -50.3289) -> (68.0301, -50.3734)
  line L1 (68.0301, -50.3734) -> (68.1013, -50.3745)
  line L2 (68.1013, -50.3745) -> (68.1738, -50.3674)
  line L3 (68.1738, -50.3674) -> (68.2469, -50.3545)
  line L4 (68.2469, -50.3545) -> (68.3205, -50.3368)
  line L5 (68.3205, -50.3368) -> (68.3945, -50.3147)
  line L6 (68.3945, -50.3147) -> (68.4687, -50.2885)
  line L7 (68.4687, -50.2885) -> (68.543, -50.2583)
  line L8 (68.543, -50.2583) -> (68.6173, -50.2244)
  line L9 (68.6173, -50.2244) -> (68.6914, -50.1869)
  line L10 (68.6914, -50.1869) -> (68.7653, -50.1458)
  line L11 (68.7653, -50.1458) -> (68.8389, -50.1012)
  line L12 (68.8389, -50.1012) -> (68.9121, -50.0532)
  line L13 (68.9121, -50.0532) -> (68.9161, -49.9236)
  line L14 (68.9161, -49.9236) -> (68.9161, -49.794)
  line L15 (68.9161, -49.794) -> (68.9121, -49.6645)
  line L16 (68.9121, -49.6645) -> (68.8389, -49.6165)
  line L17 (68.8389, -49.6165) -> (68.7653, -49.5719)
  line L18 (68.7653, -49.5719) -> (68.6914, -49.5308)
  line L19 (68.6914, -49.5308) -> (68.6173, -49.4932)
  line L20 (68.6173, -49.4932) -> (68.543, -49.4593)
  line L21 (68.543, -49.4593) -> (68.4687, -49.4292)
  line L22 (68.4687, -49.4292) -> (68.3945, -49.403)
  line L23 (68.3945, -49.403) -> (68.3205, -49.3809)
  line L24 (68.3205, -49.3809) -> (68.2469, -49.3631)
  line L25 (68.2469, -49.3631) -> (68.1738, -49.3503)
  line L26 (68.1738, -49.3503) -> (68.1013, -49.3431)
  line L27 (68.1013, -49.3431) -> (68.0301, -49.3442)
  line L28 (68.0301, -49.3442) -> (67.7406, -49.3888)
  line L29 (67.7406, -49.3888) -> (67.7105, -49.223)
  line L30 (67.7105, -49.223) -> (67.6713, -49.0591)
  line L31 (67.6713, -49.0591) -> (67.6233, -48.8975)
  line L32 (67.6233, -48.8975) -> (67.5665, -48.7389)
  line L33 (67.5665, -48.7389) -> (67.8395, -48.6327)
  line L34 (67.8395, -48.6327) -> (67.9017, -48.5981)
  line L35 (67.9017, -48.5981) -> (67.9609, -48.5557)
  line L36 (67.9609, -48.5557) -> (68.0178, -48.508)
  line L37 (68.0178, -48.508) -> (68.0727, -48.4558)
  line L38 (68.0727, -48.4558) -> (68.1257, -48.3996)
  line L39 (68.1257, -48.3996) -> (68.1768, -48.3398)
  line L40 (68.1768, -48.3398) -> (68.2261, -48.2766)
  line L41 (68.2261, -48.2766) -> (68.2734, -48.2101)
  line L42 (68.2734, -48.2101) -> (68.3189, -48.1405)
  line L43 (68.3189, -48.1405) -> (68.3623, -48.068)
  line L44 (68.3623, -48.068) -> (68.4038, -47.9925)
  line L45 (68.4038, -47.9925) -> (68.4432, -47.9144)
  line L46 (68.4432, -47.9144) -> (68.3818, -47.8002)
  line L47 (68.3818, -47.8002) -> (68.317, -47.688)
  line L48 (68.317, -47.688) -> (68.2488, -47.5777)
  line L49 (68.2488, -47.5777) -> (68.1614, -47.5728)
  line L50 (68.1614, -47.5728) -> (68.0754, -47.571)
  line L51 (68.0754, -47.571) -> (67.9908, -47.5723)
  line L52 (67.9908, -47.5723) -> (67.9079, -47.5769)
  line L53 (67.9079, -47.5769) -> (67.8266, -47.5847)
  line L54 (67.8266, -47.5847) -> (67.7472, -47.5957)
  line L55 (67.7472, -47.5957) -> (67.6698, -47.6101)
  line L56 (67.6698, -47.6101) -> (67.5947, -47.6279)
  line L57 (67.5947, -47.6279) -> (67.5221, -47.6494)
  line L58 (67.5221, -47.6494) -> (67.4523, -47.6748)
  line L59 (67.4523, -47.6748) -> (67.386, -47.7048)
  line L60 (67.386, -47.7048) -> (67.3249, -47.7414)
  line L61 (67.3249, -47.7414) -> (67.0964, -47.9247)
  line L62 (67.0964, -47.9247) -> (66.9874, -47.7962)
  line L63 (66.9874, -47.7962) -> (66.8715, -47.6739)
  line L64 (66.8715, -47.6739) -> (66.7492, -47.558)
  line L65 (66.7492, -47.558) -> (66.6207, -47.449)
  line L66 (66.6207, -47.449) -> (66.804, -47.2205)
  line L67 (66.804, -47.2205) -> (66.8406, -47.1594)
  line L68 (66.8406, -47.1594) -> (66.8706, -47.0931)
  line L69 (66.8706, -47.0931) -> (66.896, -47.0233)
  line L70 (66.896, -47.0233) -> (66.9175, -46.9507)
  line L71 (66.9175, -46.9507) -> (66.9353, -46.8756)
  line L72 (66.9353, -46.8756) -> (66.9497, -46.7982)
  line L73 (66.9497, -46.7982) -> (66.9608, -46.7188)
  line L74 (66.9608, -46.7188) -> (66.9685, -46.6376)
  line L75 (66.9685, -46.6376) -> (66.9731, -46.5546)
  line L76 (66.9731, -46.5546) -> (66.9745, -46.47)
  line L77 (66.9745, -46.47) -> (66.9726, -46.384)
  line L78 (66.9726, -46.384) -> (66.9677, -46.2966)
  line L79 (66.9677, -46.2966) -> (66.8575, -46.2284)
  line L80 (66.8575, -46.2284) -> (66.7452, -46.1636)
  line L81 (66.7452, -46.1636) -> (66.631, -46.1022)
  line L82 (66.631, -46.1022) -> (66.5529, -46.1416)
  line L83 (66.5529, -46.1416) -> (66.4775, -46.1831)
  line L84 (66.4775, -46.1831) -> (66.4049, -46.2265)
  line L85 (66.4049, -46.2265) -> (66.3353, -46.272)
  line L86 (66.3353, -46.272) -> (66.2688, -46.3193)
  line L87 (66.2688, -46.3193) -> (66.2056, -46.3686)
  line L88 (66.2056, -46.3686) -> (66.1458, -46.4197)
  line L89 (66.1458, -46.4197) -> (66.0896, -46.4727)
  line L90 (66.0896, -46.4727) -> (66.0375, -46.5276)
  line L91 (66.0375, -46.5276) -> (65.9898, -46.5846)
  line L92 (65.9898, -46.5846) -> (65.9473, -46.6437)
  line L93 (65.9473, -46.6437) -> (65.9127, -46.706)
  line L94 (65.9127, -46.706) -> (65.8065, -46.9789)
  line L95 (65.8065, -46.9789) -> (65.6479, -46.9222)
  line L96 (65.6479, -46.9222) -> (65.4863, -46.8741)
  line L97 (65.4863, -46.8741) -> (65.3224, -46.835)
  line L98 (65.3224, -46.835) -> (65.1566, -46.8048)
  line L99 (65.1566, -46.8048) -> (65.2012, -46.5153)
  line L100 (65.2012, -46.5153) -> (65.2023, -46.4441)
  line L101 (65.2023, -46.4441) -> (65.1951, -46.3716)
  line L102 (65.1951, -46.3716) -> (65.1823, -46.2985)
  line L103 (65.1823, -46.2985) -> (65.1646, -46.2249)
  line L104 (65.1646, -46.2249) -> (65.1424, -46.1509)
  line L105 (65.1424, -46.1509) -> (65.1162, -46.0767)
  line L106 (65.1162, -46.0767) -> (65.0861, -46.0024)
  line L107 (65.0861, -46.0024) -> (65.0522, -45.9282)
  line L108 (65.0522, -45.9282) -> (65.0146, -45.854)
  line L109 (65.0146, -45.854) -> (64.9735, -45.7801)
  line L110 (64.9735, -45.7801) -> (64.9289, -45.7065)
  line L111 (64.9289, -45.7065) -> (64.8809, -45.6333)
  line L112 (64.8809, -45.6333) -> (64.7514, -45.6293)
  line L113 (64.7514, -45.6293) -> (64.6218, -45.6293)
  line L114 (64.6218, -45.6293) -> (64.4922, -45.6333)
  line L115 (64.4922, -45.6333) -> (64.4442, -45.7065)
  line L116 (64.4442, -45.7065) -> (64.3996, -45.7801)
  line L117 (64.3996, -45.7801) -> (64.3585, -45.854)
  line L118 (64.3585, -45.854) -> (64.321, -45.9282)
  line L119 (64.321, -45.9282) -> (64.2871, -46.0024)
  line L120 (64.2871, -46.0024) -> (64.257, -46.0767)
  line L121 (64.257, -46.0767) -> (64.2307, -46.1509)
  line L122 (64.2307, -46.1509) -> (64.2086, -46.2249)
  line L123 (64.2086, -46.2249) -> (64.1909, -46.2985)
  line L124 (64.1909, -46.2985) -> (64.178, -46.3716)
  line L125 (64.178, -46.3716) -> (64.1709, -46.4441)
  line L126 (64.1709, -46.4441) -> (64.172, -46.5153)
  line L127 (64.172, -46.5153) -> (64.2166, -46.8048)
  line L128 (64.2166, -46.8048) -> (64.0507, -46.835)
  line L129 (64.0507, -46.835) -> (63.8868, -46.8741)
  line L130 (63.8868, -46.8741) -> (63.7253, -46.9222)
  line L131 (63.7253, -46.9222) -> (63.5666, -46.9789)
  line L132 (63.5666, -46.9789) -> (63.4605, -46.706)
  line L133 (63.4605, -46.706) -> (63.4258, -46.6437)
  line L134 (63.4258, -46.6437) -> (63.3834, -46.5846)
  line L135 (63.3834, -46.5846) -> (63.3357, -46.5276)
  line L136 (63.3357, -46.5276) -> (63.2835, -46.4727)
  line L137 (63.2835, -46.4727) -> (63.2274, -46.4197)
  line L138 (63.2274, -46.4197) -> (63.1676, -46.3686)
  line L139 (63.1676, -46.3686) -> (63.1043, -46.3193)
  line L140 (63.1043, -46.3193) -> (63.0379, -46.272)
  line L141 (63.0379, -46.272) -> (62.9683, -46.2265)
  line L142 (62.9683, -46.2265) -> (62.8957, -46.1831)
  line L143 (62.8957, -46.1831) -> (62.8203, -46.1416)
  line L144 (62.8203, -46.1416) -> (62.7421, -46.1022)
  line L145 (62.7421, -46.1022) -> (62.628, -46.1636)
  line L146 (62.628, -46.1636) -> (62.5157, -46.2284)
  line L147 (62.5157, -46.2284) -> (62.4055, -46.2966)
  line L148 (62.4055, -46.2966) -> (62.4005, -46.384)
  line L149 (62.4005, -46.384) -> (62.3987, -46.47)
  line L150 (62.3987, -46.47) -> (62.4001, -46.5546)
  line L151 (62.4001, -46.5546) -> (62.4046, -46.6376)
  line L152 (62.4046, -46.6376) -> (62.4124, -46.7188)
  line L153 (62.4124, -46.7188) -> (62.4235, -46.7982)
  line L154 (62.4235, -46.7982) -> (62.4378, -46.8756)
  line L155 (62.4378, -46.8756) -> (62.4557, -46.9507)
  line L156 (62.4557, -46.9507) -> (62.4771, -47.0233)
  line L157 (62.4771, -47.0233) -> (62.5026, -47.0931)
  line L158 (62.5026, -47.0931) -> (62.5326, -47.1594)
  line L159 (62.5326, -47.1594) -> (62.5692, -47.2205)
  line L160 (62.5692, -47.2205) -> (62.7525, -47.449)
  line L161 (62.7525, -47.449) -> (62.624, -47.558)
  line L162 (62.624, -47.558) -> (62.5016, -47.6739)
  line L163 (62.5016, -47.6739) -> (62.3858, -47.7962)
  line L164 (62.3858, -47.7962) -> (62.2767, -47.9247)
  line L165 (62.2767, -47.9247) -> (62.0483, -47.7414)
  line L166 (62.0483, -47.7414) -> (61.9872, -47.7048)
  line L167 (61.9872, -47.7048) -> (61.9209, -47.6748)
  line L168 (61.9209, -47.6748) -> (61.8511, -47.6494)
  line L169 (61.8511, -47.6494) -> (61.7785, -47.6279)
  line L170 (61.7785, -47.6279) -> (61.7033, -47.6101)
  line L171 (61.7033, -47.6101) -> (61.626, -47.5957)
  line L172 (61.626, -47.5957) -> (61.5466, -47.5847)
  line L173 (61.5466, -47.5847) -> (61.4653, -47.5769)
  line L174 (61.4653, -47.5769) -> (61.3823, -47.5723)
  line L175 (61.3823, -47.5723) -> (61.2978, -47.571)
  line L176 (61.2978, -47.571) -> (61.2117, -47.5728)
  line L177 (61.2117, -47.5728) -> (61.1243, -47.5777)
  line L178 (61.1243, -47.5777) -> (61.0561, -47.688)
  line L179 (61.0561, -47.688) -> (60.9913, -47.8002)
  line L180 (60.9913, -47.8002) -> (60.93, -47.9144)
  line L181 (60.93, -47.9144) -> (60.9694, -47.9925)
  line L182 (60.9694, -47.9925) -> (61.0108, -48.068)
  line L183 (61.0108, -48.068) -> (61.0543, -48.1405)
  line L184 (61.0543, -48.1405) -> (61.0997, -48.2101)
  line L185 (61.0997, -48.2101) -> (61.1471, -48.2766)
  line L186 (61.1471, -48.2766) -> (61.1964, -48.3398)
  line L187 (61.1964, -48.3398) -> (61.2475, -48.3996)
  line L188 (61.2475, -48.3996) -> (61.3005, -48.4558)
  line L189 (61.3005, -48.4558) -> (61.3554, -48.508)
  line L190 (61.3554, -48.508) -> (61.4123, -48.5557)
  line L191 (61.4123, -48.5557) -> (61.4715, -48.5981)
  line L192 (61.4715, -48.5981) -> (61.5337, -48.6327)
  line L193 (61.5337, -48.6327) -> (61.8067, -48.7389)
  line L194 (61.8067, -48.7389) -> (61.7499, -48.8975)
  line L195 (61.7499, -48.8975) -> (61.7019, -49.0591)
  line L196 (61.7019, -49.0591) -> (61.6627, -49.223)
  line L197 (61.6627, -49.223) -> (61.6325, -49.3888)
  line L198 (61.6325, -49.3888) -> (61.3431, -49.3442)
  line L199 (61.3431, -49.3442) -> (61.2718, -49.3431)
  line L200 (61.2718, -49.3431) -> (61.1994, -49.3503)
  line L201 (61.1994, -49.3503) -> (61.1263, -49.3631)
  line L202 (61.1263, -49.3631) -> (61.0526, -49.3809)
  line L203 (61.0526, -49.3809) -> (60.9786, -49.403)
  line L204 (60.9786, -49.403) -> (60.9045, -49.4292)
  line L205 (60.9045, -49.4292) -> (60.8302, -49.4593)
  line L206 (60.8302, -49.4593) -> (60.7559, -49.4932)
  line L207 (60.7559, -49.4932) -> (60.6818, -49.5308)
  line L208 (60.6818, -49.5308) -> (60.6079, -49.5719)
  line L209 (60.6079, -49.5719) -> (60.5342, -49.6165)
  line L210 (60.5342, -49.6165) -> (60.4611, -49.6645)
  line L211 (60.4611, -49.6645) -> (60.4571, -49.794)
  line L212 (60.4571, -49.794) -> (60.4571, -49.9236)
  line L213 (60.4571, -49.9236) -> (60.4611, -50.0532)
  line L214 (60.4611, -50.0532) -> (60.5342, -50.1012)
  line L215 (60.5342, -50.1012) -> (60.6079, -50.1458)
  line L216 (60.6079, -50.1458) -> (60.6818, -50.1869)
  line L217 (60.6818, -50.1869) -> (60.7559, -50.2244)
  line L218 (60.7559, -50.2244) -> (60.8302, -50.2583)
  line L219 (60.8302, -50.2583) -> (60.9045, -50.2885)
  line L220 (60.9045, -50.2885) -> (60.9786, -50.3147)
  line L221 (60.9786, -50.3147) -> (61.0526, -50.3368)
  line L222 (61.0526, -50.3368) -> (61.1263, -50.3545)
  line L223 (61.1263, -50.3545) -> (61.1994, -50.3674)
  line L224 (61.1994, -50.3674) -> (61.2718, -50.3745)
  line L225 (61.2718, -50.3745) -> (61.3431, -50.3734)
  line L226 (61.3431, -50.3734) -> (61.6325, -50.3289)
  line L227 (61.6325, -50.3289) -> (61.6627, -50.4947)
  line L228 (61.6627, -50.4947) -> (61.7019, -50.6586)
  line L229 (61.7019, -50.6586) -> (61.7499, -50.8201)
  line L230 (61.7499, -50.8201) -> (61.8067, -50.9788)
  line L231 (61.8067, -50.9788) -> (61.5337, -51.0849)
  line L232 (61.5337, -51.0849) -> (61.4715, -51.1196)
  line L233 (61.4715, -51.1196) -> (61.4123, -51.162)
  line L234 (61.4123, -51.162) -> (61.3554, -51.2097)
  line L235 (61.3554, -51.2097) -> (61.3005, -51.2619)
  line L236 (61.3005, -51.2619) -> (61.2475, -51.318)
  line L237 (61.2475, -51.318) -> (61.1964, -51.3778)
  line L238 (61.1964, -51.3778) -> (61.1471, -51.4411)
  line L239 (61.1471, -51.4411) -> (61.0997, -51.5076)
  line L240 (61.0997, -51.5076) -> (61.0543, -51.5771)
  line L241 (61.0543, -51.5771) -> (61.0108, -51.6497)
  line L242 (61.0108, -51.6497) -> (60.9694, -51.7251)
  line L243 (60.9694, -51.7251) -> (60.93, -51.8033)
  line L244 (60.93, -51.8033) -> (60.9913, -51.9175)
  line L245 (60.9913, -51.9175) -> (61.0561, -52.0297)
  line L246 (61.0561, -52.0297) -> (61.1243, -52.1399)
  line L247 (61.1243, -52.1399) -> (61.2117, -52.1449)
  line L248 (61.2117, -52.1449) -> (61.2978, -52.1467)
  line L249 (61.2978, -52.1467) -> (61.3823, -52.1453)
  line L250 (61.3823, -52.1453) -> (61.4653, -52.1408)
  line L251 (61.4653, -52.1408) -> (61.5466, -52.133)
  line L252 (61.5466, -52.133) -> (61.626, -52.122)
  line L253 (61.626, -52.122) -> (61.7033, -52.1076)
  line L254 (61.7033, -52.1076) -> (61.7785, -52.0898)
  line L255 (61.7785, -52.0898) -> (61.8511, -52.0683)
  line L256 (61.8511, -52.0683) -> (61.9209, -52.0429)
  line L257 (61.9209, -52.0429) -> (61.9872, -52.0128)
  line L258 (61.9872, -52.0128) -> (62.0483, -51.9762)
  line L259 (62.0483, -51.9762) -> (62.2767, -51.7929)
  line L260 (62.2767, -51.7929) -> (62.3858, -51.9214)
  line L261 (62.3858, -51.9214) -> (62.5016, -52.0438)
  line L262 (62.5016, -52.0438) -> (62.624, -52.1597)
  line L263 (62.624, -52.1597) -> (62.7525, -52.2687)
  line L264 (62.7525, -52.2687) -> (62.5692, -52.4971)
  line L265 (62.5692, -52.4971) -> (62.5326, -52.5582)
  line L266 (62.5326, -52.5582) -> (62.5026, -52.6245)
  line L267 (62.5026, -52.6245) -> (62.4771, -52.6943)
  line L268 (62.4771, -52.6943) -> (62.4557, -52.7669)
  line L269 (62.4557, -52.7669) -> (62.4378, -52.8421)
  line L270 (62.4378, -52.8421) -> (62.4235, -52.9194)
  line L271 (62.4235, -52.9194) -> (62.4124, -52.9988)
  line L272 (62.4124, -52.9988) -> (62.4046, -53.0801)
  line L273 (62.4046, -53.0801) -> (62.4001, -53.1631)
  line L274 (62.4001, -53.1631) -> (62.3987, -53.2476)
  line L275 (62.3987, -53.2476) -> (62.4005, -53.3337)
  line L276 (62.4005, -53.3337) -> (62.4055, -53.4211)
  line L277 (62.4055, -53.4211) -> (62.5157, -53.4893)
  line L278 (62.5157, -53.4893) -> (62.628, -53.5541)
  line L279 (62.628, -53.5541) -> (62.7421, -53.6154)
  line L280 (62.7421, -53.6154) -> (62.8203, -53.576)
  line L281 (62.8203, -53.576) -> (62.8957, -53.5346)
  line L282 (62.8957, -53.5346) -> (62.9683, -53.4911)
  line L283 (62.9683, -53.4911) -> (63.0379, -53.4457)
  line L284 (63.0379, -53.4457) -> (63.1043, -53.3983)
  line L285 (63.1043, -53.3983) -> (63.1676, -53.3491)
  line L286 (63.1676, -53.3491) -> (63.2274, -53.2979)
  line L287 (63.2274, -53.2979) -> (63.2835, -53.2449)
  line L288 (63.2835, -53.2449) -> (63.3357, -53.19)
  line L289 (63.3357, -53.19) -> (63.3834, -53.1331)
  line L290 (63.3834, -53.1331) -> (63.4258, -53.074)
  line L291 (63.4258, -53.074) -> (63.4605, -53.0117)
  line L292 (63.4605, -53.0117) -> (63.5666, -52.7387)
  line L293 (63.5666, -52.7387) -> (63.7253, -52.7955)
  line L294 (63.7253, -52.7955) -> (63.8868, -52.8435)
  line L295 (63.8868, -52.8435) -> (64.0507, -52.8827)
  line L296 (64.0507, -52.8827) -> (64.2166, -52.9129)
  line L297 (64.2166, -52.9129) -> (64.172, -53.2024)
  line L298 (64.172, -53.2024) -> (64.1709, -53.2736)
  line L299 (64.1709, -53.2736) -> (64.178, -53.346)
  line L300 (64.178, -53.346) -> (64.1909, -53.4192)
  line L301 (64.1909, -53.4192) -> (64.2086, -53.4928)
  line L302 (64.2086, -53.4928) -> (64.2307, -53.5668)
  line L303 (64.2307, -53.5668) -> (64.257, -53.641)
  line L304 (64.257, -53.641) -> (64.2871, -53.7152)
  line L305 (64.2871, -53.7152) -> (64.321, -53.7895)
  line L306 (64.321, -53.7895) -> (64.3585, -53.8636)